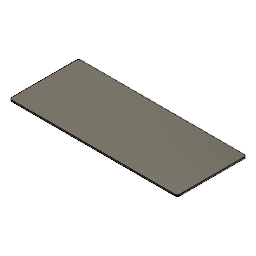
bottom (Autodesk Fusion 360 design; units mm, degrees)
Autodesk Fusion 360 part; units mm, degrees
sketch "Sketch1" plane through (0, 0, 0) normal (0, 1, 0) x (1, 0, 0)
sketch "Sketch2" plane through (0, 0, 0) normal (0, 1, 0) x (1, 0, 0)
  line L0 (0.4754, 3.1598) -> (0.339, 3.5278)
  line L1 (0.1557, 4.2912) -> (0.1102, 4.6812)
  line L2 (321.809, 133.993) -> (322.165, 133.829)
  line L3 (322.165, 133.829) -> (322.508, 133.638)
  line L4 (323.698, 1.8259) -> (323.431, 1.5379)
  line L5 (324.757, 3.9067) -> (324.651, 3.5278)
  line L6 (324.159, 2.4612) -> (323.941, 2.1346)
  line L7 (3.1805, 0.4548) -> (2.825, 0.6187)
  line L8 (4.7019, 0.0896) -> (4.3119, 0.135)
  line L9 (319.896, 134.374) -> (320.288, 134.359)
  line L10 (324.879, 4.6812) -> (324.834, 4.2912)
  line L11 (323.941, 132.314) -> (324.159, 131.987)
  line L12 (324.651, 3.5278) -> (324.514, 3.1598)
  line L13 (2.1553, 1.028) -> (1.8466, 1.2706)
  line L14 (319.896, 0.073) -> (5.0946, 0.073)
  line L15 (0.6394, 2.8043) -> (0.4754, 3.1598)
  line L16 (0.2329, 3.9067) -> (0.1557, 4.2912)
  line L17 (0.339, 3.5278) -> (0.2329, 3.9067)
  line L18 (2.825, 0.6187) -> (2.4819, 0.8103)
  line L19 (4.3119, 0.135) -> (3.9274, 0.2122)
  line L20 (324.834, 130.157) -> (324.879, 129.767)
  line L21 (1.2912, 1.8259) -> (1.0487, 2.1346)
  line L22 (322.834, 1.028) -> (322.508, 0.8103)
  line L23 (321.441, 0.3183) -> (321.062, 0.2122)
  line L24 (323.698, 132.623) -> (323.941, 132.314)
  line L25 (0.831, 2.4612) -> (0.6394, 2.8043)
  line L26 (320.288, 134.359) -> (320.678, 134.313)
  line L27 (1.8466, 1.2706) -> (1.5586, 1.5379)
  line L28 (1.5586, 1.5379) -> (1.2912, 1.8259)
  line L29 (0.0937, 5.0739) -> (0.0951, 129.374)
  line L30 (1.0487, 132.314) -> (1.2912, 132.623)
  line L31 (0.4754, 131.288) -> (0.6394, 131.644)
  line L32 (320.678, 134.313) -> (321.062, 134.236)
  line L33 (0.831, 131.987) -> (1.0487, 132.314)
  line L34 (3.9274, 134.236) -> (4.3119, 134.313)
  line L35 (324.159, 131.987) -> (324.35, 131.644)
  line L36 (3.1805, 133.993) -> (3.5485, 134.13)
  line L37 (3.9274, 0.2122) -> (3.5485, 0.3183)
  line L38 (324.514, 3.1598) -> (324.35, 2.8043)
  line L39 (324.35, 2.8043) -> (324.159, 2.4612)
  line L40 (322.508, 0.8103) -> (322.165, 0.6187)
  line L41 (5.0946, 0.073) -> (4.7019, 0.0896)
  line L42 (324.651, 130.92) -> (324.757, 130.542)
  line L43 (3.5485, 0.3183) -> (3.1805, 0.4548)
  line L44 (324.514, 131.288) -> (324.651, 130.92)
  line L45 (320.678, 0.135) -> (320.288, 0.0896)
  line L46 (1.5586, 132.91) -> (1.8466, 133.178)
  line L47 (0.1102, 4.6812) -> (0.0937, 5.0739)
  line L48 (322.508, 133.638) -> (322.834, 133.42)
  line L49 (5.0946, 134.375) -> (319.896, 134.374)
  line L50 (321.809, 0.4548) -> (321.441, 0.3183)
  line L51 (324.895, 129.374) -> (324.896, 5.0726)
  line L52 (323.431, 1.5379) -> (323.143, 1.2705)
  line L53 (322.165, 0.6187) -> (321.809, 0.4548)
  line L54 (323.941, 2.1346) -> (323.698, 1.8259)
  line L55 (324.896, 5.0726) -> (324.879, 4.6812)
  line L56 (322.834, 133.42) -> (323.143, 133.178)
  line L57 (323.431, 132.91) -> (323.698, 132.623)
  line L58 (324.35, 131.644) -> (324.514, 131.288)
  line L59 (324.757, 130.542) -> (324.834, 130.157)
  line L60 (321.062, 0.2122) -> (320.678, 0.135)
  line L61 (2.4819, 0.8103) -> (2.1553, 1.028)
  line L62 (0.1102, 129.767) -> (0.1557, 130.157)
  line L63 (321.441, 134.13) -> (321.809, 133.993)
  line L64 (324.879, 129.767) -> (324.895, 129.374)
  line L65 (1.0487, 2.1346) -> (0.831, 2.4612)
  line L66 (0.0951, 129.374) -> (0.1102, 129.767)
  line L67 (324.834, 4.2912) -> (324.757, 3.9067)
  line L68 (4.3119, 134.313) -> (4.7019, 134.359)
  line L69 (0.339, 130.92) -> (0.4754, 131.288)
  line L70 (1.2912, 132.623) -> (1.5586, 132.91)
  line L71 (0.2329, 130.542) -> (0.339, 130.92)
  line L72 (0.6394, 131.644) -> (0.831, 131.987)
  line L73 (2.4819, 133.638) -> (2.825, 133.829)
  line L74 (4.7019, 134.359) -> (5.0946, 134.375)
  line L75 (323.143, 133.178) -> (323.431, 132.91)
  line L76 (323.143, 1.2706) -> (322.834, 1.028)
  line L77 (320.288, 0.0896) -> (319.896, 0.073)
  line L78 (321.062, 134.236) -> (321.441, 134.13)
  line L79 (1.8466, 133.178) -> (2.1553, 133.42)
  line L80 (0.1557, 130.157) -> (0.2329, 130.542)
  line L81 (3.5485, 134.13) -> (3.9274, 134.236)
  line L82 (2.825, 133.829) -> (3.1805, 133.993)
  line L83 (2.1553, 133.42) -> (2.4819, 133.638)
extrude "Extrude1" add sketch "Sketch2" along normal blind 3
